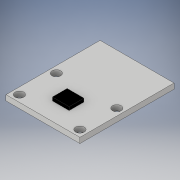
# Autodesk Inventor part: AS5047
Saved by Autodesk Inventor 2018 (Build 220112000, 112)
## iProperties
Created: 2019-11-19
Part Number: AS5047
Material: Generic
Document SubType Name: Modeling
Designer: Bunny320
Density: 1 g/cm^3
Appearance: Default
Author: Bunny320
Autodesk Inventor part; units mm, degrees
ref_plane "YZ Plane" through (0, 0, 0) normal (1, 0, 0) x (0, 1, 0)
ref_plane "XZ Plane" through (0, 0, 0) normal (0, 1, 0) x (-1, 0, 0)
ref_plane "XY Plane" through (0, 0, 0) normal (0, 0, 1) x (1, 0, 0)
sketch "Sketch1" plane through (0, 0, 0) normal (0, 0, 1) x (1, 0, 0)
  line L0 (-11, 14) -> (11, 14)
  line L1 (11, 14) -> (11, -14)
  line L2 (11, -14) -> (-11, -14)
  line L3 (-11, -14) -> (-11, 14)
  line L4 (-11, 14) -> (11, -14) construction
  line L5 (11, 14) -> (-11, -14) construction
  point P0 (0, 0)
  dimension "d0" = 22
  dimension "d1" = 28
  constraints: 12 end point, 2 midpoint, 2 parallel, 1 horizontal, 1 perpendicular
  measures "d0" distance of L0.start L0.end
  measures "d1" distance of L0.end L1.end
extrude "Extrusion1" add sketch "Sketch1" along normal blind 1.6
sketch "Sketch2" plane through (0, 0, 1.6) normal (0, 0, 1) x (1, 0, 0)
  line L0 (-9, -12) -> (9, -12)
  line L1 (9, -12) -> (9, -1)
  line L2 (9, -1) -> (-9, -1)
  line L3 (-9, -1) -> (-9, -12)
  line L4 (-9, -12) -> (9, -1) construction
  line L5 (9, -12) -> (-9, -1) construction
  line L6 (0, 19.6) -> (0, -19.6) projected
  line L7 (-11, -14) -> (11, -14) projected
  point P0 (0, 0)
  point P1 (0, -6.5)
  dimension "d4" = 11
  dimension "d5" = 18
  dimension "d6" = 2
  constraints: 12 end point, 4 coincident, 2 midpoint, 2 parallel, 1 horizontal, 1 perpendicular, 1 point on line
  measures "d4" distance of L0.end L1.end
  measures "d5" distance of L0.start L0.end
  measures "d6" distance between parallel lines of L7 L0
hole "Hole1" at (-9, -1, 1.6) at (9, -1, 1.6) at (9, -12, 1.6) at (-9, -12, 1.6) direction (0, 0, -1) diameter 2.6 end through all
sketch "Sketch3" plane through (0, 0, 1.6) normal (0, 0, 1) x (1, 0, 0)
  line L0 (-2.5, -8.7) -> (2.5, -8.7)
  line L1 (2.5, -8.7) -> (2.5, -4.3)
  line L2 (2.5, -4.3) -> (-2.5, -4.3)
  line L3 (-2.5, -4.3) -> (-2.5, -8.7)
  line L4 (-2.5, -8.7) -> (2.5, -4.3) construction
  line L5 (2.5, -8.7) -> (-2.5, -4.3) construction
  circle A0 centre (9, -1) radius 1.3 projected
  point P0 (0, 0)
  point P1 (0, -6.5)
  dimension "d14" = 5
  dimension "d15" = 4.4
  dimension "d16" = 5.5
  constraints: 12 end point, 2 midpoint, 2 parallel, 1 horizontal, 1 perpendicular, 1 vertical alignment
  measures "d14" distance of L1.end L2.end
  measures "d15" distance of L0.end L1.end
  measures "d16" vertical distance of A0.centre point (0, -6.5)
extrude "Extrusion2" add sketch "Sketch3" along normal blind 1 contours L3 L2 L1 L0
body "Solid1"
